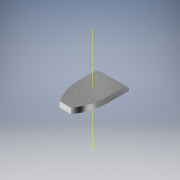
# Autodesk Inventor part: Metal Middle
Saved by Autodesk Inventor 2018 (Build 220112000, 112)
## iProperties
Created: 2017-09-12
Part Number: Metal Middle
Material: Aluminum 6061
Document SubType Name: Modeling
Designer: Rus
Density: 2.7 g/cm^3
Appearance: Aluminum - Flat
Author: Rus
Autodesk Inventor part; units mm, degrees
ref_plane "YZ Plane" through (0, 0, 0) normal (1, 0, 0) x (0, 1, 0)
ref_plane "XZ Plane" through (0, 0, 0) normal (0, 1, 0) x (-1, 0, 0)
sketch "Sketch1" plane through (0, 0, 0) normal (0, 1, 0) x (-1, 0, 0)
  line L0 (-40, 482.6) -> (-40, -482.6)
  line L1 (-40, -482.6) -> (40, -482.6)
  line L2 (40, -482.6) -> (40, 482.6)
  line L3 (40, 482.6) -> (-40, 482.6)
  line L4 (-40, 482.6) -> (40, -482.6) construction
  line L5 (-40, -482.6) -> (40, 482.6) construction
  point P0 (0, 0)
  dimension "d0" = 965.2
  dimension "d1" = 80
  constraints: 12 end point, 2 midpoint, 2 parallel, 1 perpendicular, 1 vertical
  measures "d0" distance of L0.start L0.end
  measures "d1" distance of L1.end L0.end
extrude "Extrusion1" add sketch "Sketch1" against normal blind 15.5448
ref_plane "Work Plane1" through (0, 0, 482.6) normal (1, 0, 0) x (0, 1, 0)
sketch "Sketch2" plane through (0, 0, 482.6) normal (1, 0, 0) x (0, 1, 0)
  line L0 (0, -965.2) -> (0, 0) projected
  line L1 (0, -965.2) -> (-15.5448, -965.2) projected
  line L2 (-15.5448, 0) -> (-15.5448, -965.2) projected
  line L3 (0, 0) -> (-15.5448, 0) projected
  line L4 (41.9902, -1050.1493) -> (41.9902, -1135.1493)
  line L5 (57.0671, -1050.1493) -> (57.0671, -1135.1493)
  line L6 (57.0671, -1135.1493) -> (41.9902, -1135.1493)
  line L7 (41.9902, -1092.6493) -> (57.0671, -1092.6493) construction
  line L8 (-15.5448, 0) -> (-15.5448, -965.2) construction
  line L9 (-15.5448, -965.2) -> (-15.5448, -1004.6981) construction
  line L10 (-15.5448, -1004.6981) -> (41.9902, -1021.6042) construction
  line L11 (41.9902, -1021.6042) -> (41.9902, -1050.1493) construction
  spline S0 degree 3 poles (-15.5448, -965.2) (-15.5448, -1004.6981) (41.9902, -1021.6042) (41.9902, -1050.1493) knots 1 1 1 1 2 2 2 2
  line L12 (57.0671, -1050.1493) -> (57.0671, -1021.6042) construction
  line L13 (57.0671, -1021.6042) -> (0, -1003.1803) construction
  line L14 (0, -965.2) -> (0, 0) construction
  line L15 (0, -1003.1803) -> (0, -965.2) construction
  spline S1 degree 3 poles (57.0671, -1050.1493) (57.0671, -1021.6042) (0, -1003.1803) (0, -965.2) knots 1 1 1 1 2 2 2 2
  point P0 (0, -482.6)
  dimension "d4" = 85
  dimension "d5" = 15.0769
  constraints: 8 end point, 4 vertical, 3 perpendicular, 2 equal length, 2 midpoint, 1 collinear, 1 point on line, 6 other
  measures "d4" distance of L5.start L5.end
  measures "d5" distance of L7.start L7.end
sketch "Sketch3" plane through (0, 0, 482.6) normal (1, 0, 0) x (0, 1, 0)
  line L0 (0, 0) -> (0, -965.2) projected
  line L1 (0, 0) -> (-15.5448, 0) projected
  line L2 (-15.5448, -965.2) -> (-15.5448, 0) projected
  line L3 (0, -965.2) -> (-15.5448, -965.2) projected
  arc A0 (2.1293, 48.5593) -> (-15.5448, 0) centre (60, 0) ccw
  arc A1 (14.0373, 38.5673) -> (0, 0) centre (60, 0) ccw
  line L4 (2.1293, 48.5593) -> (18.199, 67.7104)
  line L5 (0, 0) -> (-15.5448, 0) construction
  line L6 (2.1293, 48.5593) -> (14.0373, 38.5673) construction
  line L7 (14.0373, 38.5673) -> (30.107, 57.7184)
  arc A2 (18.199, 67.7104) -> (32.2363, 106.2776) centre (-27.7637, 106.2776) ccw
  arc A3 (30.107, 57.7184) -> (47.7811, 106.2776) centre (-27.7637, 106.2776) ccw
  line L8 (32.2363, 106.2776) -> (32.2363, 233.2776)
  line L9 (32.2363, 233.2776) -> (47.7811, 233.2776)
  line L10 (47.7811, 233.2776) -> (47.7811, 106.2776)
  line L11 (30.107, 57.7184) -> (18.199, 67.7104) construction
  line L12 (32.2363, 106.2776) -> (47.7811, 106.2776) construction
  point P0 (0, -482.6)
  dimension "d17" = 127
  dimension "d18" = 140
  dimension "d19" = 60
  dimension "d21" = 140
  dimension "d22" = 25
  constraints: 16 end point, 8 point on circle, 7 tangent, 6 coincident, 4 centre point, 4 equal length, 2 line through centre, 2 perpendicular, 1 equal radius
  measures "d17" distance of L9.end L10.end
  measures "d18" angle of L7 L0
  measures "d19" radius of A1
  measures "d21" angle of L4 L8
  measures "d22" distance of L11.start point (14.037, 38.567)
extrude "Extrusion2" add sketch "Sketch3" along normal up to surface (80 mm away) from surface at -40 contours L1 A0 L4 A2 L8 L9 L10 A3 L7 A1
sketch "Sketch9" plane through (-40, 47.7811, 588.8776) normal (0, 1, 0) x (1, 0, 0)
  line L0 (0, -127) -> (0, 0) construction
  line L1 (0, 0) -> (0, -127) construction
  line L2 (80, -127) -> (80, 0) construction
  line L3 (0, -127) -> (0, -49.1262)
  line L4 (80, 0) -> (80, -127) projected
  line L5 (80, -49.1262) -> (80, -127)
  arc A0 (0, -49.1262) -> (24.125, -127) centre (137.7482, -49.1262) ccw
  arc A1 (55.875, -127) -> (80, -49.1262) centre (-57.7482, -49.1262) ccw
  line L6 (24.125, -127) -> (55.875, -127)
  line L7 (0, -127) -> (80, -127) projected
  line L8 (55.875, -127) -> (80, -127)
  line L9 (80, -127) -> (80, -49.1262)
  line L10 (0, -127) -> (24.125, -127)
  line L11 (55.875, -127) -> (80, -127)
  line L12 (24.125, -127) -> (0, -127)
  point P0 (40, 588.8776)
  dimension "d41" = 31.75
  constraints: 16 end point, 4 collinear, 4 point on circle, 2 centre point, 2 point on line, 2 tangent, 1 equal radius, 1 horizontal, 1 perpendicular
  measures "d41" distance of L6.start L6.end
sketch "Sketch10" plane through (-40, 47.7811, 588.8776) normal (0, 1, 0) x (1, 0, 0)
  line L0 (11.425, -92.075) -> (68.575, -92.075) construction
  line L1 (68.575, -92.075) -> (68.575, -12.7) construction
  line L2 (68.575, -12.7) -> (11.425, -12.7) construction
  line L3 (11.425, -12.7) -> (11.425, -92.075) construction
  line L4 (11.425, -92.075) -> (68.575, -12.7) construction
  line L5 (68.575, -92.075) -> (11.425, -12.7) construction
  line L6 (12.6315, -90.043) -> (67.3685, -90.043)
  line L7 (67.3685, -90.043) -> (67.3685, -14.732)
  line L8 (67.3685, -14.732) -> (12.6315, -14.732)
  line L9 (12.6315, -14.732) -> (12.6315, -90.043)
  line L10 (12.6315, -90.043) -> (67.3685, -14.732) construction
  line L11 (67.3685, -90.043) -> (12.6315, -14.732) construction
  line L12 (18.965, -84.1375) -> (61.035, -84.1375) construction
  line L13 (61.035, -84.1375) -> (61.035, -20.6375) construction
  line L14 (61.035, -20.6375) -> (18.965, -20.6375) construction
  line L15 (18.965, -20.6375) -> (18.965, -84.1375) construction
  line L16 (18.965, -84.1375) -> (61.035, -20.6375) construction
  line L17 (61.035, -84.1375) -> (18.965, -20.6375) construction
  line L18 (18.965, -84.1375) -> (61.035, -84.1375) construction
  line L19 (61.035, -84.1375) -> (61.035, -74.6125) construction
  line L20 (61.035, -74.6125) -> (18.965, -74.6125) construction
  line L21 (18.965, -74.6125) -> (18.965, -84.1375) construction
  line L22 (68.575, -12.7) -> (80, -12.7) construction
  line L23 (11.425, -12.7) -> (0, -12.7) construction
  line L24 (0, -127) -> (0, 0) construction
  line L25 (80, -127) -> (80, 0) projected
  line L26 (0, 0) -> (80, 0) projected
  point P0 (40, 588.8776)
  point P1 (40, -52.3875)
  dimension "d33" = 57.15
  dimension "d34" = 79.375
  dimension "d35" = 54.737
  dimension "d36" = 75.311
  dimension "d37" = 42.07
  dimension "d38" = 63.5
  dimension "d39" = 9.525
  dimension "d40" = 12.7
  constraints: 48 end point, 8 parallel, 6 coincident, 6 horizontal, 6 midpoint, 4 perpendicular, 2 point on line, 1 collinear
  measures "d33" distance of L0.start L0.end
  measures "d34" distance of L1.end L0.end
  measures "d35" distance of L6.start L6.end
  measures "d36" distance of L7.end L6.end
  measures "d37" distance of L12.start L12.end
  measures "d38" distance of L13.end L12.end
  measures "d39" distance of L19.end L12.end
  measures "d40" distance between parallel lines of L2 L26
extrude "Extrusion7" cut sketch "Sketch9" against normal through all
hole "Hole1" at (-21.035, 47.7811, 673.0151) at (-21.035, 47.7811, 663.4901) at (21.035, 47.7811, 673.0151) at (21.035, 47.7811, 663.4901) at (21.035, 47.7811, 609.5151) at (-21.035, 47.7811, 609.5151) direction (0, -1, 0) diameter 4.7625 end through all
sketch "Sketch11" plane through (-40, 32.2363, 588.8776) normal (0, -1, 0) x (1, 0, 0)
  line L0 (11.425, 92.075) -> (68.575, 92.075) construction
  line L1 (11.425, 12.7) -> (11.425, 92.075) construction
  line L2 (68.575, 92.075) -> (68.575, 12.7) construction
  line L3 (11.425, 12.7) -> (68.575, 12.7)
  line L4 (68.575, 12.7) -> (68.575, 92.075)
  line L5 (68.575, 92.075) -> (11.425, 92.075)
  line L6 (11.425, 92.075) -> (11.425, 12.7)
  line L7 (11.425, 12.7) -> (68.575, 92.075) construction
  line L8 (68.575, 12.7) -> (11.425, 92.075) construction
  point P0 (40, -588.8776)
  point P1 (40, 52.3875)
  constraints: 12 end point, 2 midpoint, 2 parallel, 1 horizontal, 1 perpendicular
extrude "Extrusion8" cut sketch "Sketch11" against normal blind 3
sketch "Sketch12" plane through (-40, 47.7811, 588.8776) normal (0, 1, 0) x (1, 0, 0)
  line L0 (80, -127) -> (0, -127)
  line L1 (0, -127) -> (0, 0)
  line L2 (0, 0) -> (80, 0)
  line L3 (80, 0) -> (80, -127)
  line L4 (24.125, -127) -> (55.875, -127) projected
  line L5 (0, 0) -> (0, -49.1262) projected
  point P0 (40, 588.8776)
  constraints: 8 end point, 2 parallel, 2 point on line, 1 coincident, 1 horizontal, 1 perpendicular
extrude "Extrusion9" cut sketch "Sketch12" against normal through all keep common part
sketch "Sketch13" plane through (40, 32.2363, 638.0038) normal (1, 0, 0) x (0, 0, -1)
  line L0 (49.1262, 15.5448) -> (49.1262, 0) projected
  line L1 (0, 15.5448) -> (49.1262, 15.5448) projected
  line L2 (0, 0) -> (0, 15.5448) projected
  line L3 (49.1262, 0) -> (0, 0) projected
  line L4 (26.1074, 3) -> (26.1074, 15.5448) projected
  line L5 (30.8699, 3) -> (30.8699, 15.5448) projected
  line L6 (-42.9488, 3) -> (36.4262, 3) projected
  line L7 (36.4262, 0) -> (36.4262, 3) projected
  line L8 (49.1262, 0) -> (59.1262, 0)
  line L9 (59.1262, 0) -> (59.1262, 7.7724)
  line L10 (59.1262, 7.7724) -> (49.1262, 7.7724)
  line L11 (49.1262, 7.7724) -> (49.1262, 0)
  line L12 (49.1262, 15.5448) -> (39.1262, 15.5448)
  line L13 (39.1262, 15.5448) -> (39.1262, 7.7724)
  line L14 (39.1262, 7.7724) -> (49.1262, 7.7724)
  line L15 (49.1262, 7.7724) -> (49.1262, 15.5448)
  line L16 (39.1262, 15.5448) -> (49.1262, 7.7724)
  line L17 (49.1262, 0) -> (49.1262, 15.5448) projected
  line L18 (39.1262, 15.5448) -> (49.1262, 15.5448)
  point P0 (638.0038, -32.2363)
  dimension "d58" = 10
  constraints: 20 end point, 4 parallel, 2 equal length, 2 horizontal, 2 perpendicular, 1 collinear
  measures "d58" distance of L10.end L9.end
extrude "Extrusion10" add sketch "Sketch13" against normal up to surface (80 mm away) contours L10 L9 L8 L0
body "Solid1"
